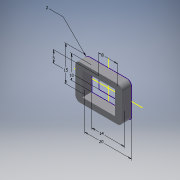
# Autodesk Inventor part: slab
Saved by Autodesk Inventor 2018 (Build 220112000, 112)
## iProperties
Created: 2018-12-04
Part Number: slab
Material: Generic
Document SubType Name: Modeling
Designer: Jerry
Density: 1 g/cm^3
Appearance: Default
Author: Jerry
Autodesk Inventor part; units mm, degrees
ref_plane "YZ Plane" through (0, 0, 0) normal (1, 0, 0) x (0, 1, 0)
ref_plane "XZ Plane" through (0, 0, 0) normal (0, 1, 0) x (-1, 0, 0)
ref_plane "XY Plane" through (0, 0, 0) normal (0, 0, 1) x (1, 0, 0)
sketch "Sketch1" plane through (0, 0, 0) normal (0, 1, 0) x (-1, 0, 0)
  line L0 (-14.5799, 0) -> (14.5799, 0) projected
  line L1 (7, 5) -> (-7, 5)
  line L2 (-7, 5) -> (-7, -5)
  line L3 (-7, -5) -> (7, -5)
  line L4 (7, -5) -> (7, 5)
  line L5 (8, 7.5) -> (-8, 7.5)
  line L6 (-10, 5.5) -> (-10, -5.5)
  line L7 (-8, -7.5) -> (8, -7.5)
  line L8 (10, -5.5) -> (10, 5.5)
  line L9 (0, -11.0799) -> (0, 11.0799) projected
  arc A0 (10, 5.5) -> (8, 7.5) centre (8, 5.5) ccw
  arc A1 (8, -7.5) -> (10, -5.5) centre (8, -5.5) ccw
  arc A2 (-10, -5.5) -> (-8, -7.5) centre (-8, -5.5) ccw
  arc A3 (-8, 7.5) -> (-10, 5.5) centre (-8, 5.5) ccw
  line L10 (-4, 2.5) -> (4, 2.5)
  line L11 (4, 2.5) -> (4, -2.5)
  line L12 (4, -2.5) -> (-4, -2.5)
  line L13 (-4, -2.5) -> (-4, 2.5)
  point P0 (0, 0)
  point P1 (10, 7.5)
  point P2 (10, -7.5)
  dimension "d0" = 10
  dimension "d1" = 15
  dimension "d2" = 14
  dimension "d3" = 20
  dimension "d4" = 2
  dimension "d9" = 5
  dimension "d10" = 8
  constraints: 24 end point, 8 point on circle, 8 tangent, 6 parallel, 4 centre point, 4 point on line, 3 equal radius, 3 horizontal, 3 perpendicular, 6 other
  measures "d0" distance of L3.end L1.start
  measures "d1" distance of point (10, -7.5) point (10, 7.5)
  measures "d2" distance between parallel lines of L2 L4
  measures "d3" distance between parallel lines of L6 L8
  measures "d4" radius of A0
  measures "d9" distance of L10.end L11.end
  measures "d10" distance of L10.start L10.end
extrude "Extrusion1" add sketch "Sketch1" against normal blind 4 contours L6 A3 L5 L9 L1 L2 L0 | L0 L2 L3 L9 L7 A2 L6 | L9 L5 A0 L8 L0 L4 L1 | L3 L4 L0 L8 A1 L7 L9
body "Solid1"
